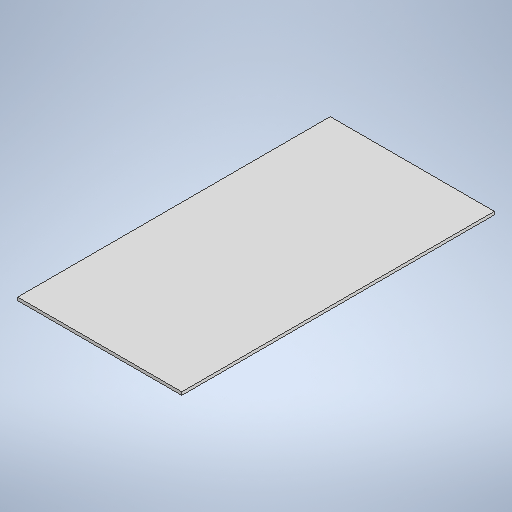
# Autodesk Inventor part: Mega
Saved by Autodesk Inventor 2025.1 (Build 291241000, 241)
## iProperties
Created: 2025-05-15
Part Number: Mega
Material: Generic
Document SubType Name: Modeling
Designer: asus
Density: 1 g/cm^3
Appearance: Default
Author: asus
Autodesk Inventor part; units mm, degrees
ref_plane "YZ Plane" through (0, 0, 0) normal (1, 0, 0) x (0, 1, 0)
ref_plane "XZ Plane" through (0, 0, 0) normal (0, 1, 0) x (-1, 0, 0)
ref_plane "XY Plane" through (0, 0, 0) normal (0, 0, 1) x (1, 0, 0)
sketch "Sketch1" plane through (0, 0, 0) normal (0, 1, 0) x (-1, 0, 0)
  line L0 (0, 0) -> (53.3, 0)
  line L1 (53.3, 0) -> (53.3, -101.52)
  line L2 (53.3, -101.52) -> (0, -101.52)
  line L3 (0, -101.52) -> (0, 0)
  dimension "d0" = 101.52
  dimension "d1" = 53.3
  constraints: 8 end point, 2 parallel, 1 horizontal, 1 perpendicular
  measures "d0" distance of L0.end L1.end
  measures "d1" distance of L1.end L2.end
extrude "Extrusion1" add sketch "Sketch1" along normal blind 1
body "Solid1"
